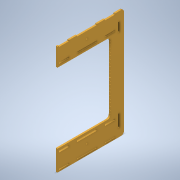
# Autodesk Inventor part: side bracer
Saved by Autodesk Inventor 2022 (Build 260153000, 153)
## iProperties
Created: 2021-05-28
Part Number: side bracer
Material: Brass, Soft Yellow
Document SubType Name: Modeling
Designer: benka
Density: 8.47 g/cm^3
Appearance: Brass - Satin
Author: benka
Autodesk Inventor part; units mm, degrees
ref_plane "YZ Plane" through (0, 0, 0) normal (1, 0, 0) x (0, 1, 0)
ref_plane "XZ Plane" through (0, 0, 0) normal (0, 1, 0) x (-1, 0, 0)
ref_plane "XY Plane" through (0, 0, 0) normal (0, 0, 1) x (1, 0, 0)
sketch "Sketch1" plane through (0, 0, 0) normal (1, 0, 0) x (0, 1, 0)
  line L0 (-181.221, 115.0382) -> (-181.221, -87.4618)
  line L1 (-171.221, -97.4618) -> (156.7524, -97.4618)
  line L2 (166.7524, -67.9618) -> (166.7524, -87.4618)
  circle A0 centre (141.7569, 21.2887) radius 2
  line L3 (-117.2477, 115.0382) -> (-181.221, 115.0382)
  line L4 (-117.2477, 115.0382) -> (-115.2203, 115.0382)
  line L5 (-115.2203, 115.0382) -> (-115.2203, -43.8573)
  arc A1 (-115.2203, -43.8573) -> (-105.2478, -53.8299) centre (-105.2478, -43.8573) ccw
  line L6 (108.7524, -43.8299) -> (108.7524, 115.0382)
  line L7 (108.7524, 115.0382) -> (166.7524, 115.0382)
  arc A2 (98.7524, -53.8299) -> (108.7524, -43.8299) centre (98.7524, -43.8299) ccw
  arc A3 (156.7524, -97.4618) -> (166.7524, -87.4618) centre (156.7524, -87.4618) ccw
  arc A4 (-181.221, -87.4618) -> (-171.221, -97.4618) centre (-171.221, -87.4618) ccw
  circle A5 centre (-148.2261, 21.2878) radius 2
  line L8 (108.7565, -82.9618) -> (138.0065, -82.9618) projected
  line L9 (138.0065, -82.9618) -> (138.0065, -77.9618) projected
  line L10 (108.7565, -77.9618) -> (138.0065, -77.9618) projected
  line L11 (108.7565, -82.9618) -> (108.7565, -77.9618) projected
  line L12 (-155.2435, -82.9618) -> (-115.2435, -82.9618) projected
  line L13 (-115.2435, -82.9618) -> (-115.2435, -77.9618) projected
  line L14 (-155.2435, -77.9618) -> (-115.2435, -77.9618) projected
  line L15 (-155.2435, -82.9618) -> (-155.2435, -77.9618) projected
  line L16 (-173.221, -67.9618) -> (-173.221, -36.7118) projected
  line L17 (-173.221, -36.7118) -> (-176.221, -36.7118) projected
  line L18 (-176.221, -67.9618) -> (-176.221, -36.7118) projected
  line L19 (-173.221, -67.9618) -> (-176.221, -67.9618) projected
  line L20 (-173.221, -10.4618) -> (-173.221, 52.5382) projected
  line L21 (-173.221, 52.5382) -> (-176.221, 52.5382) projected
  line L22 (-176.221, -10.4618) -> (-176.221, 52.5382) projected
  line L23 (-173.221, -10.4618) -> (-176.221, -10.4618) projected
  line L24 (-173.221, 78.7882) -> (-173.221, 110.0382) projected
  line L25 (-173.221, 110.0382) -> (-176.221, 110.0382) projected
  line L26 (-176.221, 78.7882) -> (-176.221, 110.0382) projected
  line L27 (-173.221, 78.7882) -> (-176.221, 78.7882) projected
  line L28 (-128.2203, 110.0382) -> (-128.2203, 78.7882) projected
  line L29 (-128.2203, 78.7882) -> (-123.2203, 78.7882) projected
  line L30 (-123.2203, 110.0382) -> (-123.2203, 78.7882) projected
  line L31 (-128.2203, 110.0382) -> (-123.2203, 110.0382) projected
  line L32 (-128.2203, 52.5382) -> (-128.2203, -10.4618) projected
  line L33 (-128.2203, -10.4618) -> (-123.2203, -10.4618) projected
  line L34 (-123.2203, 52.5382) -> (-123.2203, -10.4618) projected
  line L35 (-128.2203, 52.5382) -> (-123.2203, 52.5382) projected
  line L36 (-128.2203, -36.7118) -> (-128.2203, -67.9618) projected
  line L37 (-128.2203, -67.9618) -> (-123.2203, -67.9618) projected
  line L38 (-123.2203, -36.7118) -> (-123.2203, -67.9618) projected
  line L39 (-128.2203, -36.7118) -> (-123.2203, -36.7118) projected
  line L40 (121.7524, -67.9618) -> (121.7524, -36.7118) projected
  line L41 (121.7524, -36.7118) -> (116.7524, -36.7118) projected
  line L42 (116.7524, -67.9618) -> (116.7524, -36.7118) projected
  line L43 (121.7524, -67.9618) -> (116.7524, -67.9618) projected
  line L44 (121.7524, -10.4618) -> (121.7524, 52.5382) projected
  line L45 (121.7524, 52.5382) -> (116.7524, 52.5382) projected
  line L46 (116.7524, -10.4618) -> (116.7524, 52.5382) projected
  line L47 (121.7524, -10.4618) -> (116.7524, -10.4618) projected
  line L48 (121.7524, 78.7882) -> (121.7524, 110.0382) projected
  line L49 (121.7524, 110.0382) -> (116.7524, 110.0382) projected
  line L50 (116.7524, 78.7882) -> (116.7524, 110.0382) projected
  line L51 (121.7524, 78.7882) -> (116.7524, 78.7882) projected
  line L52 (163.7524, -67.9618) -> (166.7524, -67.9618)
  line L53 (163.7524, -67.9618) -> (163.7524, -36.7118)
  line L54 (163.7524, -36.7118) -> (166.7524, -36.7118)
  line L55 (166.7524, -36.7118) -> (166.7524, -10.4618)
  line L56 (163.7524, -10.4618) -> (166.7524, -10.4618)
  line L57 (163.7524, -10.4618) -> (163.7524, 52.5382)
  line L58 (163.7524, 52.5382) -> (166.7524, 52.5382)
  line L59 (166.7524, 52.5382) -> (166.7524, 78.7882)
  line L60 (163.7524, 78.7882) -> (166.7524, 78.7882)
  line L61 (163.7524, 78.7882) -> (163.7524, 110.0382)
  line L62 (166.7524, 110.0382) -> (166.7524, 115.0382)
  line L63 (163.7524, 110.0382) -> (166.7524, 110.0382)
  line L64 (108.7524, 58.4483) -> (-3.2341, 58.4483) construction
  arc A6 (-4.2477, -53.8299) -> (-2.2477, -53.8299) centre (-3.2477, -53.8299) ccw
  line L65 (6.7523, -51.2048) -> (6.7523, -55.8299) construction
  line L66 (7.0023, -55.8299) -> (7.0023, -53.8299)
  line L67 (7.0023, -55.8299) -> (6.5023, -55.8299)
  line L68 (6.5023, -55.8299) -> (6.5023, -53.8299)
  line L69 (-3.2477, -53.8299) -> (-3.2477, -37.0259) construction
  line L70 (16.5023, -55.8299) -> (16.5023, -53.8299)
  line L71 (17.0023, -55.8299) -> (16.5023, -55.8299)
  line L72 (17.0023, -55.8299) -> (17.0023, -53.8299)
  line L73 (26.5023, -55.8299) -> (26.5023, -53.8299)
  line L74 (27.0023, -55.8299) -> (26.5023, -55.8299)
  line L75 (27.0023, -55.8299) -> (27.0023, -53.8299)
  line L76 (36.5023, -55.8299) -> (36.5023, -53.8299)
  line L77 (37.0023, -55.8299) -> (36.5023, -55.8299)
  line L78 (37.0023, -55.8299) -> (37.0023, -53.8299)
  line L79 (46.5023, -55.8299) -> (46.5023, -53.8299)
  line L80 (47.0023, -55.8299) -> (46.5023, -55.8299)
  line L81 (47.0023, -55.8299) -> (47.0023, -53.8299)
  line L82 (56.5023, -55.8299) -> (56.5023, -53.8299)
  line L83 (57.0023, -55.8299) -> (56.5023, -55.8299)
  line L84 (57.0023, -55.8299) -> (57.0023, -53.8299)
  line L85 (66.5023, -55.8299) -> (66.5023, -53.8299)
  line L86 (67.0023, -55.8299) -> (66.5023, -55.8299)
  line L87 (67.0023, -55.8299) -> (67.0023, -53.8299)
  line L88 (76.5023, -55.8299) -> (76.5023, -53.8299)
  line L89 (77.0023, -55.8299) -> (76.5023, -55.8299)
  line L90 (77.0023, -55.8299) -> (77.0023, -53.8299)
  line L91 (67.0023, -53.8299) -> (76.5023, -53.8299)
  line L92 (57.0023, -53.8299) -> (66.5023, -53.8299)
  line L93 (56.5023, -53.8299) -> (47.0023, -53.8299)
  line L94 (46.5023, -53.8299) -> (37.0023, -53.8299)
  line L95 (36.5023, -53.8299) -> (27.0023, -53.8299)
  line L96 (26.5023, -53.8299) -> (17.0023, -53.8299)
  line L97 (16.5023, -53.8299) -> (7.0023, -53.8299)
  line L98 (-2.2477, -53.8299) -> (6.5023, -53.8299)
  line L99 (6.7523, -55.8299) -> (6.7523, -57.8299)
  line L100 (6.7523, -57.8299) -> (6.7523, -58.8299) construction
  line L101 (16.7523, -55.8299) -> (16.7523, -57.8299)
  line L102 (16.7523, -57.8299) -> (16.7523, -58.8299) construction
  line L103 (26.7523, -55.8299) -> (26.7523, -57.8299)
  line L104 (26.7523, -57.8299) -> (26.7523, -58.8299) construction
  line L105 (36.7523, -55.8299) -> (36.7523, -57.8299)
  line L106 (36.7523, -57.8299) -> (36.7523, -58.8299) construction
  line L107 (46.7523, -55.8299) -> (46.7523, -57.8299)
  line L108 (46.7523, -57.8299) -> (46.7523, -58.8299) construction
  line L109 (56.7523, -55.8299) -> (56.7523, -57.8299)
  line L110 (56.7523, -57.8299) -> (56.7523, -58.8299) construction
  line L111 (66.7523, -55.8299) -> (66.7523, -57.8299)
  line L112 (66.7523, -57.8299) -> (66.7523, -58.8299) construction
  line L113 (76.7523, -55.8299) -> (76.7523, -57.8299)
  line L114 (76.7523, -57.8299) -> (76.7523, -58.8299) construction
  line L115 (-3.2477, -57.8299) -> (-3.2477, -58.8299) construction
  line L116 (-3.2477, -57.8299) -> (-3.2477, -54.8299)
  line L117 (86.5023, -55.8299) -> (86.5023, -53.8299)
  line L118 (87.0023, -55.8299) -> (86.5023, -55.8299)
  line L119 (87.0023, -55.8299) -> (87.0023, -53.8299)
  line L120 (77.0023, -53.8299) -> (86.5023, -53.8299)
  line L121 (86.7523, -57.8299) -> (86.7523, -58.8299) construction
  line L122 (86.7523, -55.8299) -> (86.7523, -57.8299)
  line L123 (96.5023, -55.8299) -> (96.5023, -53.8299)
  line L124 (97.0023, -55.8299) -> (96.5023, -55.8299)
  line L125 (97.0023, -55.8299) -> (97.0023, -53.8299)
  line L126 (87.0023, -53.8299) -> (96.5023, -53.8299)
  line L127 (96.7523, -57.8299) -> (96.7523, -58.8299) construction
  line L128 (96.7523, -55.8299) -> (96.7523, -57.8299)
  line L129 (97.0023, -53.8299) -> (98.7524, -53.8299)
  line L130 (-13.2477, -51.2048) -> (-13.2477, -55.8299) construction
  line L131 (-13.4977, -55.8299) -> (-13.4977, -53.8299)
  line L132 (-13.4977, -55.8299) -> (-12.9977, -55.8299)
  line L133 (-12.9977, -55.8299) -> (-12.9977, -53.8299)
  line L134 (-22.9977, -55.8299) -> (-22.9977, -53.8299)
  line L135 (-23.4977, -55.8299) -> (-22.9977, -55.8299)
  line L136 (-23.4977, -55.8299) -> (-23.4977, -53.8299)
  line L137 (-32.9977, -55.8299) -> (-32.9977, -53.8299)
  line L138 (-33.4977, -55.8299) -> (-32.9977, -55.8299)
  line L139 (-33.4977, -55.8299) -> (-33.4977, -53.8299)
  line L140 (-42.9977, -55.8299) -> (-42.9977, -53.8299)
  line L141 (-43.4977, -55.8299) -> (-42.9977, -55.8299)
  line L142 (-43.4977, -55.8299) -> (-43.4977, -53.8299)
  line L143 (-52.9977, -55.8299) -> (-52.9977, -53.8299)
  line L144 (-53.4977, -55.8299) -> (-52.9977, -55.8299)
  line L145 (-53.4977, -55.8299) -> (-53.4977, -53.8299)
  line L146 (-62.9977, -55.8299) -> (-62.9977, -53.8299)
  line L147 (-63.4977, -55.8299) -> (-62.9977, -55.8299)
  line L148 (-63.4977, -55.8299) -> (-63.4977, -53.8299)
  line L149 (-72.9977, -55.8299) -> (-72.9977, -53.8299)
  line L150 (-73.4977, -55.8299) -> (-72.9977, -55.8299)
  line L151 (-73.4977, -55.8299) -> (-73.4977, -53.8299)
  line L152 (-82.9977, -55.8299) -> (-82.9977, -53.8299)
  line L153 (-83.4977, -55.8299) -> (-82.9977, -55.8299)
  line L154 (-83.4977, -55.8299) -> (-83.4977, -53.8299)
  line L155 (-73.4977, -53.8299) -> (-82.9977, -53.8299)
  line L156 (-63.4977, -53.8299) -> (-72.9977, -53.8299)
  line L157 (-62.9977, -53.8299) -> (-53.4977, -53.8299)
  line L158 (-52.9977, -53.8299) -> (-43.4977, -53.8299)
  line L159 (-42.9977, -53.8299) -> (-33.4977, -53.8299)
  line L160 (-32.9977, -53.8299) -> (-23.4977, -53.8299)
  line L161 (-22.9977, -53.8299) -> (-13.4977, -53.8299)
  line L162 (-4.2477, -53.8299) -> (-12.9977, -53.8299)
  line L163 (-13.2477, -55.8299) -> (-13.2477, -57.8299)
  line L164 (-13.2477, -57.8299) -> (-13.2477, -58.8299) construction
  line L165 (-23.2477, -57.8299) -> (-23.2477, -58.8299) construction
  line L166 (-23.2477, -55.8299) -> (-23.2477, -57.8299)
  line L167 (-33.2477, -57.8299) -> (-33.2477, -58.8299) construction
  line L168 (-33.2477, -55.8299) -> (-33.2477, -57.8299)
  line L169 (-43.2477, -57.8299) -> (-43.2477, -58.8299) construction
  line L170 (-43.2477, -55.8299) -> (-43.2477, -57.8299)
  line L171 (-53.2477, -57.8299) -> (-53.2477, -58.8299) construction
  line L172 (-53.2477, -55.8299) -> (-53.2477, -57.8299)
  line L173 (-63.2477, -57.8299) -> (-63.2477, -58.8299) construction
  line L174 (-63.2477, -55.8299) -> (-63.2477, -57.8299)
  line L175 (-73.2477, -57.8299) -> (-73.2477, -58.8299) construction
  line L176 (-73.2477, -55.8299) -> (-73.2477, -57.8299)
  line L177 (-83.2477, -57.8299) -> (-83.2477, -58.8299) construction
  line L178 (-83.2477, -55.8299) -> (-83.2477, -57.8299)
  line L179 (-83.4977, -53.8299) -> (-92.9977, -53.8299)
  line L180 (-93.2477, -57.8299) -> (-93.2477, -58.8299) construction
  line L181 (-93.4977, -55.8299) -> (-92.9977, -55.8299)
  line L182 (-92.9977, -55.8299) -> (-92.9977, -53.8299)
  line L183 (-93.4977, -55.8299) -> (-93.4977, -53.8299)
  line L184 (-93.2477, -55.8299) -> (-93.2477, -57.8299)
  line L185 (-93.4977, -53.8299) -> (-102.9977, -53.8299)
  line L186 (-103.2477, -57.8299) -> (-103.2477, -58.8299) construction
  line L187 (-103.4977, -55.8299) -> (-102.9977, -55.8299)
  line L188 (-102.9977, -55.8299) -> (-102.9977, -53.8299)
  line L189 (-103.4977, -55.8299) -> (-103.4977, -53.8299)
  line L190 (-103.2477, -55.8299) -> (-103.2477, -57.8299)
  line L191 (-103.4977, -53.8299) -> (-105.2478, -53.8299)
  line L192 (-93.2477, -57.8299) -> (-93.2477, -58.8299) construction
  line L193 (-83.2477, -57.8299) -> (-83.2477, -58.8299) construction
  line L194 (-73.2477, -57.8299) -> (-73.2477, -58.8299) construction
  line L195 (-63.2477, -57.8299) -> (-63.2477, -58.8299) construction
  line L196 (-53.2477, -57.8299) -> (-53.2477, -58.8299) construction
  line L197 (-43.2477, -57.8299) -> (-43.2477, -58.8299) construction
  line L198 (-33.2477, -57.8299) -> (-33.2477, -58.8299) construction
  line L199 (-23.2477, -57.8299) -> (-23.2477, -58.8299) construction
  line L200 (-103.2477, -57.8299) -> (-103.2477, -58.8299) construction
  line L201 (-13.2477, -57.8299) -> (-13.2477, -58.8299) construction
  line L202 (-3.2477, -57.8299) -> (-3.2477, -58.8299) construction
  point P0 (141.7524, 19.2994)
  point P1 (166.7524, -92.4608)
  point P2 (161.7524, -97.4618)
  point P3 (-176.2435, -97.4618)
  point P4 (-181.221, -92.4608)
  point P5 (-115.2203, -34.9618)
  dimension "d34" = 10
  dimension "d35" = 10
  dimension "d40" = 212.5
  dimension "d41" = 212.5
  dimension "d44" = 4
  dimension "d50" = 8
  dimension "d51" = 8
  dimension "d52" = 223.9727
  dimension "d53" = 5
  dimension "d54" = 45.0007
  dimension "d55" = 3
  dimension "d56" = 5
  dimension "d57" = 5
  dimension "d58" = 42
  dimension "d59" = 3
  dimension "d60" = 111.9865
  dimension "d61" = 2
  dimension "d81" = 2
  dimension "d82" = 10
  dimension "d85" = 10
  dimension "d91" = 2
  dimension "d92" = 1
  dimension "d97" = 2
  dimension "d98" = 1
  dimension "d103" = 2
  dimension "d104" = 1
  dimension "d109" = 2
  dimension "d110" = 1
  dimension "d115" = 2
  dimension "d116" = 1
  dimension "d121" = 2
  dimension "d122" = 1
  dimension "d127" = 2
  dimension "d128" = 1
  dimension "d133" = 2
  dimension "d134" = 1
  dimension "d140" = 1
  dimension "d145" = 2
  dimension "d146" = 1
  dimension "d151" = 2
  dimension "d152" = 1
  dimension "d159" = 1
  dimension "d160" = 1
  dimension "d161" = 1
  dimension "d162" = 1
  dimension "d163" = 1
  dimension "d164" = 1
  dimension "d165" = 1
  dimension "d166" = 1
  dimension "d167" = 1
  dimension "d168" = 1
  dimension "d169" = 1
  constraints: 318 end point, 73 symmetric about line, 63 vertical, 13 horizontal, 11 point on circle, 7 centre point, 7 collinear, 7 point on line, 6 tangent, 3 perpendicular, 2 coincident, 2 parallel, 1 equal radius, 63 other
  measures "d34" radius of A2
  measures "d35" radius of A3
  measures "d40" distance between parallel lines of L1 L7
  measures "d41" distance between parallel lines of L1 L3
  measures "d44" diameter of A5
  measures "d50" distance between parallel lines of L5 L30
  measures "d51" distance between parallel lines of L6 L50
  measures "d52" distance between parallel lines of L5 L6
  measures "d53" distance between parallel lines of L28 L30
  measures "d54" distance between parallel lines of L24 L28
  measures "d55" distance between parallel lines of L26 L24
  measures "d56" distance between parallel lines of L0 L26
  measures "d57" distance between parallel lines of L48 L50
  measures "d58" distance between parallel lines of L61 L48
  measures "d59" distance between parallel lines of L61 L62
  measures "d60" distance of L64.start L64.end
  measures "d61" diameter of A6
  measures "d81" distance of L66.start L66.end
  measures "d82" distance between parallel lines of L65 L69
  measures "d85" distance of L67.end L70.start
  measures "d91" distance of L65.end L99.end
  measures "d92" distance of L99.end L100.end
  measures "d97" distance of L101.start L102.start
  measures "d98" distance of L102.start L102.end
  measures "d103" distance of L103.start L104.start
  measures "d104" distance of L104.start L104.end
  measures "d109" distance of L105.start L106.start
  measures "d110" distance of L106.start L106.end
  measures "d115" distance of L107.start L108.start
  measures "d116" distance of L108.start L108.end
  measures "d121" distance of L109.start L110.start
  measures "d122" distance of L110.start L110.end
  measures "d127" distance of L111.start L112.start
  measures "d128" distance of L112.start L112.end
  measures "d133" distance of L113.start L114.start
  measures "d134" distance of L114.start L114.end
  measures "d140" distance of L115.start L115.end
  measures "d145" distance of L122.start L121.start
  measures "d146" distance of L121.start L121.end
  measures "d151" distance of L128.start L127.start
  measures "d152" distance of L127.start L127.end
  measures "d159" distance of L184.end L192.end
  measures "d160" distance of L177.start L193.end
  measures "d161" distance of L194.start L175.end
  measures "d162" distance of L195.start L173.end
  measures "d163" distance of L196.start L171.end
  measures "d164" distance of L169.start L197.end
  measures "d165" distance of L168.end L198.end
  measures "d166" distance of L166.end L199.end
  measures "d167" distance of L200.start L186.end
  measures "d168" distance of L163.end L201.end
  measures "d169" distance of L115.start L202.end
extrude "Extrusion1" add sketch "Sketch1" along normal blind 5
body "Solid1"
